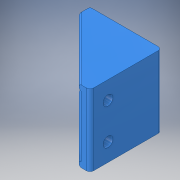
# Autodesk Inventor part: 90deg_4040
Saved by Autodesk Inventor 2019.4 (Build 234330000, 330)
## iProperties
Created: 2021-02-06
Part Number: 90deg_4040
Material: ABS Plastic
Document SubType Name: Modeling
Designer: Jorian Brusind
Density: 1.06 g/cm^3
Appearance: Cyan
Author: Jorian Brusind
Autodesk Inventor part; units mm, degrees
ref_plane "YZ Plane" through (0, 0, 0) normal (1, 0, 0) x (0, 1, 0)
ref_plane "XZ Plane" through (0, 0, 0) normal (0, 1, 0) x (-1, 0, 0)
ref_plane "XY Plane" through (0, 0, 0) normal (0, 0, 1) x (1, 0, 0)
sketch "Sketch1" plane through (0, 0, 0) normal (0, 1, 0) x (-1, 0, 0)
  line L0 (0, 0) -> (0, -34)
  line L1 (0, 0) -> (34, 0) construction
  line L2 (0, -34) -> (34, -34)
  line L3 (0, 0) -> (-6, 0)
  line L4 (-6, 0) -> (-6, -40)
  line L5 (-6, -40) -> (34, -40)
  line L6 (34, -40) -> (34, -34)
  dimension "d0" = 34
  dimension "d1" = 90
  dimension "d2" = 34
  dimension "d3" = 90
  dimension "d4" = 6
  dimension "d5" = 40
  constraints: 14 end point, 4 perpendicular, 3 horizontal, 1 vertical
  measures "d0" distance of L0.start L0.end
  measures "d1" angle of L0 L1
  measures "d2" distance of L0.end L2.end
  measures "d3" angle of L2 L0
  measures "d4" distance of L0.start L3.end
  measures "d5" distance of L3.end L4.end
extrude "Extrusion1" add sketch "Sketch1" along normal blind 40
sketch "Sketch2" plane through (-34, 0, -34) normal (0, 0, 1) x (1, 0, 0)
  circle A0 centre (10, 10) radius 2.75
  line L0 (0, 0) -> (0, 40) projected
  line L1 (34, 0) -> (0, 0) projected
  circle A1 centre (10, 30.5) radius 2.75
  dimension "d8" = 5.5
  dimension "d9" = 10
  dimension "d10" = 10
  dimension "d43" = 5.5
  dimension "d44" = 15
  dimension "d45" = 10
  constraints: 2 centre point
  measures "d8" diameter of A0
  measures "d9" distance from line of L0 A0.centre
  measures "d10" distance from line of L1 A0.centre
  measures "d43" diameter of A1
  measures "d45" distance from line of L0 A1.centre
sketch "Sketch3" plane through (0, 0, -34) normal (-1, 0, 0) x (0, 0, 1)
  circle A0 centre (24, 10) radius 2.75
  line L0 (34, 0) -> (34, 40) projected
  line L1 (34, 0) -> (0, 0) projected
  circle A1 centre (24, 30) radius 2.75
  dimension "d21" = 5.5
  dimension "d22" = 10
  dimension "d23" = 10
  dimension "d46" = 5.5
  dimension "d47" = 20
  dimension "d48" = 10
  constraints: 2 centre point
  measures "d21" diameter of A0
  measures "d22" distance from line of L0 A0.centre
  measures "d23" distance from line of L1 A0.centre
  measures "d46" diameter of A1
  measures "d47" distance of A0.centre A1.centre
  measures "d48" distance from line of L0 A1.centre
sketch "Sketch4" plane through (0, 40, 0) normal (0, 1, 0) x (1, 0, 0)
  line L0 (-34, 34) -> (0, 34) projected
  line L1 (0, 0) -> (-34, 34)
  line L2 (-34, 34) -> (0, 34)
  line L3 (0, 34) -> (0, 0)
  constraints: 6 end point, 1 collinear, 1 perpendicular
extrude "Extrusion4" add sketch "Sketch4" against normal blind 3
sketch "Sketch5" plane through (0, 0, 0) normal (0, -1, 0) x (1, 0, 0)
  line L0 (0, -34) -> (-34, -34) projected
  line L1 (0, 0) -> (0, -34) projected
  line L2 (-34, -34) -> (0, 0)
  line L3 (0, 0) -> (0, -34)
  line L4 (0, -34) -> (-34, -34)
  constraints: 6 end point, 1 collinear, 1 perpendicular, 1 point on line
extrude "Extrusion5" add sketch "Sketch5" against normal blind 3
fillet "Fillet1" radius 1 6 edges at (-17, 0, -17) (-17, 3, -17) (-17, 37, -17) (-17, 40, -17) (-34, 20, -34) (-34, 20, -40)
fillet "Fillet2" radius 1 3 edges at (0, 37.5, 0) (0, 20, 0) (0, 2.5, 0)
fillet "Fillet3" radius 2 1 edges at (6, 20, -40)
fillet "Fillet4" radius 2 1 edges at (6, 20, 0)
extrude "Extrusion6" cut sketch "Sketch2" against normal blind 6
extrude "Extrusion7" cut sketch "Sketch3" against normal blind 6
body "Solid1"
